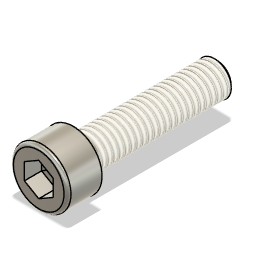
EchoWeather_SupportRod (Autodesk Fusion 360 archive; units mm, degrees)
design "Broached Hexagon Socket Head Cap Screw ASME B18.3.1M - M6x1 x 25 Steel Grade 2 Plain"
description: Broached Hexagon Socket Head Cap Screw ASME B18.3.1M - M6x1 x 25
part number: BSHCS ASME B18.3.1M - M6x1 x 25 Steel Grade 2 Plain
Autodesk Fusion 360 part; units mm, degrees
sketch "Sketch1" plane through (0, 0, 0) normal (0, 1, 0) x (1, 0, 0)
  line L0 (-3, 0) -> (-3, 25)
  line L1 (-3, 25) -> (0, 25)
  line L2 (0, 25) -> (0, -6)
  line L3 (-3, 0) -> (-5, 0)
  line L4 (-5, 0) -> (-5, -6)
  line L5 (-5, -6) -> (0, -6)
  dimension "d9" = 6
  dimension "d66" = 10
  dimension "d101" = 25
  dimension "d102" = 6
  constraint perpendicular L0 L1
  constraint collinear origin L1.end L2.end
  constraint perpendicular L0 L3
  constraint coincident origin L3
  constraint vertical L0
  constraint vertical L2
  constraint parallel L2 L4
  constraint coincident L2 L5.end
  constraint perpendicular L2 L5
  measures "d101" distance of origin L1
  measures "d102" distance of L3.end L5
revolve "Revolve1" add sketch "Sketch1" angle 360 about axis through (0, 0, -25) along (0, 0, 1)
ref_plane "WorkPlane1" through (0, 0, 6) normal (0, 0, 1) x (1, 0, 0)
sketch "Sketch6" plane through (0, 0, 6) normal (0, 0, 1) x (1, 0, 0)
  line L0 (-2.5, 0) -> (2.5, 0) construction
  line L1 (0, 0) -> (-2.5, 1.4434)
  line L2 (-2.5, -1.4434) -> (-2.5, 1.4434)
  line L3 (-2.5, -1.4434) -> (0, 0)
  dimension "d100" = 150
  dimension "d103" = 5
  constraint horizontal L0
  constraint midpoint L1.start L0
  constraint coincident L1.start L3.end
  constraint perpendicular L0 L2
  constraint midpoint L0.start L2
  constraint coincident L1.end L2.end
  measures "d100" angle of L0 L1
  measures "d103" distance of L0.end L2
extrude "Extrude1" cut sketch "Sketch6" against normal blind 3
pattern_circular "C-Pattern1" count 6 over 360 about axis through (0, 0, 1.75) along (0, 0, 1) of "Extrude1"
extrude "Extrude2" cut 1 faces at (0.8333, -0.4811, 3) along direction (0, 0, -1) blind 3 draft -85
thread "Thread3" "ANSI Metric M Profile 6.0 M6x1 M6x1 4g6g" major diameter 5.884 minor diameter 4.764 pitch 1 angle 60 resizes the face on face at (-2.9963, 0.1495, -8.3333) from (0, 0, -1.8269) to (0, 0, -25)
fillet "Fillet4" radius 0.6 1 edges at (-4.6616, 1.8081, 6)
sketch "Sketch7" plane through (0, 0, 0) normal (0, 1, 0) x (1, 0, 0)
  line L0 (-3.06, 25) -> (-3.06, 24.3866)
  line L1 (-3.06, 24.3866) -> (-2.3866, 25)
  line L2 (0, 25) -> (0, -6)
  line L3 (-3.06, 25) -> (0, 25)
  dimension "d104" = 2.3866
  dimension "d105" = 3.06
  dimension "d106" = 0.6135
  constraint coincident L2.start L3.end
  constraint perpendicular L2 L3
  constraint coincident L1.end L3
  constraint perpendicular L0 L3
  measures "d104" distance of L1.end L2
  measures "d105" distance of L0 L2.start
  measures "d106" distance of L0.end L3
revolve "Revolve3" cut sketch "Sketch7" angle 360 about axis through (0, 0, 1.75) along (0, 0, 1)
equation "d9 = adsk_nomdia"
equation "adsk_nomlen = 25.00 mm"
equation "adsk_headh = 6.00 mm"
equation "adsk_headdia = 10.00 mm"
equation "adsk_nomdia = 6.00 mm"
equation "adsk_philwidth = 5.00 mm"
equation "d31 = -adsk_phildepth"
equation "adsk_phildepth = 3.00 mm"
equation "d66 = adsk_headdia"
equation "d71 = adsk_headh"
equation "d76 = -adsk_phildepth"
equation "adsk_thrlen = 23.1731 mm"
equation "d86 = adsk_nomdia * 0.1"
equation "adsk_startlen = 0.61345 mm"
equation "adsk_endpointdia = 4.7731 mm"
equation "d101 = adsk_nomlen"
equation "d102 = adsk_headh"
equation "d103 = adsk_philwidth"
equation "d104 = adsk_endpointdia / 2"
equation "d105 = adsk_nomdia * 0.51"
equation "d106 = adsk_startlen"
equation "d108 = min(adsk_thrlen; adsk_nomlen - 0.001 mm)"
